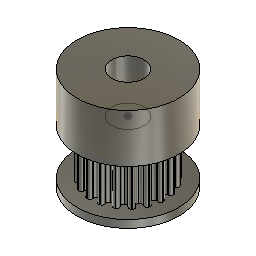
drive gear, 5mm shaft, 20 teeth v7 (Autodesk Fusion 360 design; units mm, degrees)
Autodesk Fusion 360 part; units mm, degrees
sketch "Sketch1" plane through (0, 0, 0) normal (0, 0, 1) x (1, 0, 0) in component "drive gear, 5mm shaft, 20 teeth"
  circle A0 centre (-19.8485, 10.6997) radius 8
  circle A1 centre (-19.8485, 10.6997) radius 2.5
  line L0 (-19.8485, 10.6997) -> (-14.5702, 12.4148) construction
  line L1 (-19.8485, 10.6997) -> (-14.7985, 10.6997) construction
  line L2 (-14.8275, 11.0683) -> (-14.8317, 11.1211)
  line L3 (-14.4955, 11.5475) -> (-14.3004, 11.5784)
  line L4 (-14.5702, 12.4148) -> (-14.5062, 12.4355)
  line L5 (-14.4288, 10.6997) -> (-14.2985, 10.6997)
  line L6 (-13.974, 12.0669) -> (-13.9936, 12.1485)
  arc A2 (-14.4955, 11.5475) -> (-14.8317, 11.1211) centre (-14.4329, 11.1525) ccw
  arc A3 (-14.8275, 11.0683) -> (-14.4288, 10.6997) centre (-14.4288, 11.0997) ccw
  arc A4 (-13.9936, 12.1485) -> (-14.5062, 12.4355) centre (-14.3826, 12.0551) ccw
  arc A5 (-14.3004, 11.5784) -> (-13.974, 12.0669) centre (-14.363, 11.9735) ccw
  line L7 (-14.694, 12.3745) -> (-14.5702, 12.4148)
  arc A6 (-15.1872, 12.6019) -> (-14.694, 12.3745) centre (-14.8176, 12.7549) ccw
  line L8 (-15.1872, 12.6019) -> (-15.2074, 12.6507)
  arc A7 (-15.0195, 13.1602) -> (-15.2074, 12.6507) centre (-14.8379, 12.8038) ccw
  line L9 (-15.0195, 13.1602) -> (-14.8435, 13.2499)
  arc A8 (-14.8435, 13.2499) -> (-14.684, 13.8153) centre (-15.0251, 13.6063) ccw
  line L10 (-14.684, 13.8153) -> (-14.7279, 13.8869)
  arc A9 (-14.7279, 13.8869) -> (-15.304, 14.0015) centre (-15.0689, 13.6779) ccw
  line L11 (-15.3585, 13.9619) -> (-15.304, 14.0015)
  line L12 (-15.4638, 13.8854) -> (-15.3585, 13.9619)
  arc A10 (-16.0031, 13.9492) -> (-15.4638, 13.8854) centre (-15.699, 14.209) ccw
  line L13 (-16.0031, 13.9492) -> (-16.0375, 13.9894)
  arc A11 (-16.0162, 14.5321) -> (-16.0375, 13.9894) centre (-15.7333, 14.2492) ccw
  line L14 (-16.0162, 14.5321) -> (-15.8765, 14.6717)
  arc A12 (-15.8765, 14.6717) -> (-15.8996, 15.2587) centre (-16.1593, 14.9546) ccw
  line L15 (-15.8996, 15.2587) -> (-15.9634, 15.3132)
  arc A13 (-15.9634, 15.3132) -> (-16.5468, 15.2442) centre (-16.2232, 15.0091) ccw
  line L16 (-16.5863, 15.1898) -> (-16.5468, 15.2442)
  line L17 (-16.6629, 15.0844) -> (-16.5863, 15.1898)
  arc A14 (-17.1955, 14.9784) -> (-16.6629, 15.0844) centre (-16.9865, 15.3195) ccw
  line L18 (-17.1955, 14.9784) -> (-17.2406, 15.0061)
  arc A15 (-17.388, 15.5287) -> (-17.2406, 15.0061) centre (-17.0316, 15.3471) ccw
  line L19 (-17.388, 15.5287) -> (-17.2983, 15.7047)
  arc A16 (-17.2983, 15.7047) -> (-17.5017, 16.2559) centre (-17.6547, 15.8863) ccw
  line L20 (-17.5017, 16.2559) -> (-17.5792, 16.288)
  arc A17 (-17.5792, 16.288) -> (-18.1127, 16.0421) centre (-17.7323, 15.9185) ccw
  line L21 (-18.1335, 15.9781) -> (-18.1127, 16.0421)
  line L22 (-18.1737, 15.8542) -> (-18.1335, 15.9781)
  arc A18 (-18.6475, 15.5889) -> (-18.1737, 15.8542) centre (-18.5541, 15.9778) ccw
  line L23 (-18.6475, 15.5889) -> (-18.699, 15.6012)
  arc A19 (-19.0007, 16.0527) -> (-18.699, 15.6012) centre (-18.6056, 15.9902) ccw
  line L24 (-19.0007, 16.0527) -> (-18.9698, 16.2478)
  arc A20 (-18.9698, 16.2478) -> (-19.3335, 16.7092) centre (-19.3649, 16.3104) ccw
  line L25 (-19.3335, 16.7092) -> (-19.4171, 16.7158)
  arc A21 (-19.4171, 16.7158) -> (-19.8485, 16.317) centre (-19.4485, 16.317) ccw
  line L26 (-19.8485, 16.2497) -> (-19.8485, 16.317)
  line L27 (-19.8485, 16.1195) -> (-19.8485, 16.2497)
  arc A22 (-20.2171, 15.7207) -> (-19.8485, 16.1195) centre (-20.2485, 16.1195) ccw
  line L28 (-20.2171, 15.7207) -> (-20.2699, 15.7165)
  arc A23 (-20.6964, 16.0527) -> (-20.2699, 15.7165) centre (-20.3013, 16.1153) ccw
  line L29 (-20.6964, 16.0527) -> (-20.7273, 16.2478)
  arc A24 (-20.7273, 16.2478) -> (-21.2157, 16.5742) centre (-21.1223, 16.1853) ccw
  line L30 (-21.2157, 16.5742) -> (-21.2973, 16.5546)
  arc A25 (-21.2973, 16.5546) -> (-21.5844, 16.0421) centre (-21.2039, 16.1657) ccw
  line L31 (-21.5636, 15.9781) -> (-21.5844, 16.0421)
  line L32 (-21.5233, 15.8542) -> (-21.5636, 15.9781)
  arc A26 (-21.7507, 15.361) -> (-21.5233, 15.8542) centre (-21.9037, 15.7306) ccw
  line L33 (-21.7507, 15.361) -> (-21.7996, 15.3408)
  arc A27 (-22.309, 15.5287) -> (-21.7996, 15.3408) centre (-21.9526, 15.7103) ccw
  line L34 (-22.309, 15.5287) -> (-22.3987, 15.7047)
  arc A28 (-22.3987, 15.7047) -> (-22.9641, 15.8642) centre (-22.7551, 15.5231) ccw
  line L35 (-22.9641, 15.8642) -> (-23.0357, 15.8204)
  arc A29 (-23.0357, 15.8204) -> (-23.1503, 15.2442) centre (-22.8267, 15.4793) ccw
  line L36 (-23.1107, 15.1898) -> (-23.1503, 15.2442)
  line L37 (-23.0342, 15.0844) -> (-23.1107, 15.1898)
  arc A30 (-23.098, 14.5451) -> (-23.0342, 15.0844) centre (-23.3578, 14.8493) ccw
  line L38 (-23.098, 14.5451) -> (-23.1382, 14.5107)
  arc A31 (-23.6809, 14.5321) -> (-23.1382, 14.5107) centre (-23.398, 14.8149) ccw
  line L39 (-23.6809, 14.5321) -> (-23.8205, 14.6717)
  arc A32 (-23.8205, 14.6717) -> (-24.4075, 14.6487) centre (-24.1034, 14.3889) ccw
  line L40 (-24.4075, 14.6487) -> (-24.462, 14.5848)
  arc A33 (-24.462, 14.5848) -> (-24.393, 14.0015) centre (-24.1579, 14.3251) ccw
  line L41 (-24.3386, 13.9619) -> (-24.393, 14.0015)
  line L42 (-24.2332, 13.8854) -> (-24.3386, 13.9619)
  arc A34 (-24.1272, 13.3528) -> (-24.2332, 13.8854) centre (-24.4683, 13.5618) ccw
  line L43 (-24.1272, 13.3528) -> (-24.1549, 13.3076)
  arc A35 (-24.6776, 13.1602) -> (-24.1549, 13.3076) centre (-24.496, 13.5166) ccw
  line L44 (-24.6776, 13.1602) -> (-24.8536, 13.2499)
  arc A36 (-24.8536, 13.2499) -> (-25.4047, 13.0466) centre (-25.0351, 12.8935) ccw
  line L45 (-25.4047, 13.0466) -> (-25.4368, 12.969)
  arc A37 (-25.4368, 12.969) -> (-25.1909, 12.4355) centre (-25.0673, 12.816) ccw
  line L46 (-25.1269, 12.4148) -> (-25.1909, 12.4355)
  line L47 (-25.003, 12.3745) -> (-25.1269, 12.4148)
  arc A38 (-24.7377, 11.9007) -> (-25.003, 12.3745) centre (-25.1266, 11.9941) ccw
  line L48 (-24.7377, 11.9007) -> (-24.75, 11.8492)
  arc A39 (-25.2015, 11.5475) -> (-24.75, 11.8492) centre (-25.139, 11.9426) ccw
  line L49 (-25.2015, 11.5475) -> (-25.3966, 11.5784)
  arc A40 (-25.3966, 11.5784) -> (-25.858, 11.2148) centre (-25.4592, 11.1834) ccw
  line L50 (-25.858, 11.2148) -> (-25.8646, 11.1311)
  arc A41 (-25.8646, 11.1311) -> (-25.4658, 10.6997) centre (-25.4658, 11.0997) ccw
  line L51 (-25.3985, 10.6997) -> (-25.4658, 10.6997)
  line L52 (-25.2683, 10.6997) -> (-25.3985, 10.6997)
  arc A42 (-24.8695, 10.3311) -> (-25.2683, 10.6997) centre (-25.2683, 10.2997) ccw
  line L53 (-24.8695, 10.3311) -> (-24.8654, 10.2783)
  arc A43 (-25.2015, 9.8519) -> (-24.8654, 10.2783) centre (-25.2641, 10.2469) ccw
  line L54 (-25.2015, 9.8519) -> (-25.3966, 9.821)
  arc A44 (-25.3966, 9.821) -> (-25.723, 9.3325) centre (-25.3341, 9.4259) ccw
  line L55 (-25.723, 9.3325) -> (-25.7034, 9.2509)
  arc A45 (-25.7034, 9.2509) -> (-25.1909, 8.9639) centre (-25.3145, 9.3443) ccw
  line L56 (-25.1269, 8.9847) -> (-25.1909, 8.9639)
  line L57 (-25.003, 9.0249) -> (-25.1269, 8.9847)
  arc A46 (-24.5099, 8.7976) -> (-25.003, 9.0249) centre (-24.8794, 8.6445) ccw
  line L58 (-24.5099, 8.7976) -> (-24.4896, 8.7487)
  arc A47 (-24.6776, 8.2392) -> (-24.4896, 8.7487) centre (-24.8592, 8.5956) ccw
  line L59 (-24.6776, 8.2392) -> (-24.8536, 8.1495)
  arc A48 (-24.8536, 8.1495) -> (-25.013, 7.5841) centre (-24.672, 7.7931) ccw
  line L60 (-25.013, 7.5841) -> (-24.9692, 7.5126)
  arc A49 (-24.9692, 7.5126) -> (-24.393, 7.398) centre (-24.6281, 7.7216) ccw
  line L61 (-24.3386, 7.4375) -> (-24.393, 7.398)
  line L62 (-24.2332, 7.5141) -> (-24.3386, 7.4375)
  arc A50 (-23.6939, 7.4502) -> (-24.2332, 7.5141) centre (-23.9981, 7.1904) ccw
  line L63 (-23.6939, 7.4502) -> (-23.6595, 7.41)
  arc A51 (-23.6809, 6.8674) -> (-23.6595, 7.41) centre (-23.9637, 7.1502) ccw
  line L64 (-23.6809, 6.8674) -> (-23.8205, 6.7277)
  arc A52 (-23.8205, 6.7277) -> (-23.7975, 6.1407) centre (-23.5377, 6.4448) ccw
  line L65 (-23.7975, 6.1407) -> (-23.7337, 6.0862)
  arc A53 (-23.7337, 6.0862) -> (-23.1503, 6.1552) centre (-23.4739, 6.3903) ccw
  line L66 (-23.1107, 6.2097) -> (-23.1503, 6.1552)
  line L67 (-23.0342, 6.315) -> (-23.1107, 6.2097)
  arc A54 (-22.5016, 6.421) -> (-23.0342, 6.315) centre (-22.7106, 6.0799) ccw
  line L68 (-22.5016, 6.421) -> (-22.4564, 6.3933)
  arc A55 (-22.309, 5.8707) -> (-22.4564, 6.3933) centre (-22.6654, 6.0523) ccw
  line L69 (-22.309, 5.8707) -> (-22.3987, 5.6947)
  arc A56 (-22.3987, 5.6947) -> (-22.1954, 5.1435) centre (-22.0423, 5.5131) ccw
  line L70 (-22.1954, 5.1435) -> (-22.1178, 5.1114)
  arc A57 (-22.1178, 5.1114) -> (-21.5844, 5.3574) centre (-21.9648, 5.481) ccw
  line L71 (-21.5636, 5.4213) -> (-21.5844, 5.3574)
  line L72 (-21.5233, 5.5452) -> (-21.5636, 5.4213)
  arc A58 (-21.0495, 5.8106) -> (-21.5233, 5.5452) centre (-21.1429, 5.4216) ccw
  line L73 (-21.0495, 5.8106) -> (-20.9981, 5.7982)
  arc A59 (-20.6964, 5.3467) -> (-20.9981, 5.7982) centre (-21.0914, 5.4092) ccw
  line L74 (-20.6964, 5.3467) -> (-20.7273, 5.1516)
  arc A60 (-20.7273, 5.1516) -> (-20.3636, 4.6902) centre (-20.3322, 5.089) ccw
  line L75 (-20.3636, 4.6902) -> (-20.2799, 4.6837)
  arc A61 (-20.2799, 4.6837) -> (-19.8485, 5.0824) centre (-20.2485, 5.0824) ccw
  line L76 (-19.8485, 5.1497) -> (-19.8485, 5.0824)
  line L77 (-19.8485, 5.2799) -> (-19.8485, 5.1497)
  arc A62 (-19.4799, 5.6787) -> (-19.8485, 5.2799) centre (-19.4485, 5.2799) ccw
  line L78 (-19.4799, 5.6787) -> (-19.4271, 5.6829)
  arc A63 (-19.0007, 5.3467) -> (-19.4271, 5.6829) centre (-19.3958, 5.2841) ccw
  line L79 (-19.0007, 5.3467) -> (-18.9698, 5.1516)
  arc A64 (-18.9698, 5.1516) -> (-18.4813, 4.8252) centre (-18.5747, 5.2142) ccw
  line L80 (-18.4813, 4.8252) -> (-18.3997, 4.8448)
  arc A65 (-18.3997, 4.8448) -> (-18.1127, 5.3574) centre (-18.4931, 5.2337) ccw
  line L81 (-18.1335, 5.4213) -> (-18.1127, 5.3574)
  line L82 (-18.1737, 5.5452) -> (-18.1335, 5.4213)
  arc A66 (-17.9464, 6.0384) -> (-18.1737, 5.5452) centre (-17.7933, 5.6688) ccw
  line L83 (-17.9464, 6.0384) -> (-17.8975, 6.0586)
  arc A67 (-17.388, 5.8707) -> (-17.8975, 6.0586) centre (-17.7444, 5.6891) ccw
  line L84 (-17.388, 5.8707) -> (-17.2983, 5.6947)
  arc A68 (-17.2983, 5.6947) -> (-16.7329, 5.5352) centre (-16.9419, 5.8763) ccw
  line L85 (-16.7329, 5.5352) -> (-16.6614, 5.5791)
  arc A69 (-16.6614, 5.5791) -> (-16.5468, 6.1552) centre (-16.8704, 5.9201) ccw
  line L86 (-16.5863, 6.2097) -> (-16.5468, 6.1552)
  line L87 (-16.6629, 6.315) -> (-16.5863, 6.2097)
  arc A70 (-16.599, 6.8543) -> (-16.6629, 6.315) centre (-16.3393, 6.5501) ccw
  line L88 (-16.599, 6.8543) -> (-16.5588, 6.8887)
  arc A71 (-16.0162, 6.8674) -> (-16.5588, 6.8887) centre (-16.299, 6.5845) ccw
  line L89 (-16.0162, 6.8674) -> (-15.8765, 6.7277)
  arc A72 (-15.8765, 6.7277) -> (-15.2895, 6.7508) centre (-15.5937, 7.0105) ccw
  line L90 (-15.2895, 6.7508) -> (-15.235, 6.8146)
  arc A73 (-15.235, 6.8146) -> (-15.304, 7.398) centre (-15.5392, 7.0743) ccw
  line L91 (-15.3585, 7.4375) -> (-15.304, 7.398)
  line L92 (-15.4638, 7.5141) -> (-15.3585, 7.4375)
  arc A74 (-15.5698, 8.0467) -> (-15.4638, 7.5141) centre (-15.2287, 7.8377) ccw
  line L93 (-15.5698, 8.0467) -> (-15.5421, 8.0918)
  arc A75 (-15.0195, 8.2392) -> (-15.5421, 8.0918) centre (-15.2011, 7.8828) ccw
  line L94 (-15.0195, 8.2392) -> (-14.8435, 8.1495)
  arc A76 (-14.8435, 8.1495) -> (-14.2923, 8.3528) centre (-14.6619, 8.5059) ccw
  line L95 (-14.2923, 8.3528) -> (-14.2602, 8.4304)
  arc A77 (-14.2602, 8.4304) -> (-14.5062, 8.9639) centre (-14.6298, 8.5834) ccw
  line L96 (-14.5702, 8.9847) -> (-14.5062, 8.9639)
  line L97 (-14.694, 9.0249) -> (-14.5702, 8.9847)
  arc A78 (-14.9594, 9.4987) -> (-14.694, 9.0249) centre (-14.5704, 9.4053) ccw
  line L98 (-14.9594, 9.4987) -> (-14.947, 9.5502)
  arc A79 (-14.4955, 9.8519) -> (-14.947, 9.5502) centre (-14.5581, 9.4568) ccw
  line L99 (-14.4955, 9.8519) -> (-14.3004, 9.821)
  arc A80 (-14.3004, 9.821) -> (-13.8391, 10.1847) centre (-14.2378, 10.216) ccw
  line L100 (-13.8391, 10.1847) -> (-13.8325, 10.2683)
  arc A81 (-13.8325, 10.2683) -> (-14.2312, 10.6997) centre (-14.2312, 10.2997) ccw
  line L101 (-14.2985, 10.6997) -> (-14.2312, 10.6997)
  dimension "d6_1_1" = 16
  dimension "d8_1_1" = 5
  dimension "d1_1" = 18
  dimension "d19_1" = 5.55
  dimension "d20_1" = 5.05
  dimension "d22_1" = 0.5
  dimension "d24_1" = 0.4
  dimension "d25_1" = 0.4
  dimension "d26_1" = 0.4
  dimension "d27_1" = 0.4
  dimension "d29_1" = 360
  constraint concentric A0 A1
  constraint horizontal L1
  constraint parallel L0 L4
  constraint coincident A0.centre A1.centre
  constraint parallel L1 L5
  constraint tangent L3 A2
  constraint tangent L2 A3
  constraint tangent L6 A4
  constraint tangent L3 A5
  constraint tangent L4 A4
  constraint tangent L6 A5
  constraint tangent L2 A2
  constraint tangent L5 A3
  measures "d6_1_1" diameter of A0
  measures "d8_1_1" diameter of A1
  measures "d1_1" angle of L0 L1
  measures "d19_1" distance of A0.centre L0.end
  measures "d20_1" distance of A0.centre L1.end
  measures "d22_1" distance of L1.end L5.end
  measures "d24_1" radius of A3
  measures "d25_1" radius of A2
  measures "d26_1" radius of A5
  measures "d27_1" radius of A4
extrude "Extrude1" add sketch "Sketch1" along normal mid plane 9.65 contours A0 | L2 L3 L4 L5 L6 A2 A3 A4 A5 L7 A6 L8 A7 L9 A8 L10 A9 L11 L12 A10 L13 A11 L14 A12 L15 A13 L16 L17 A14 L18 A15 L19 A16 L20 A17 L21 L22 A18 L23 A19 L24 A20 L25 A21 L26 L27 A22 L28 A23 L29 A24 L30 A25 L31 L32 A26 L33 A27 L34 A28 L35 A29 L36 L37 A30 L38 A31 L39 A32 L40 A33 L41 L42 A34 L43 A35 L44 A36 L45 A37 L46 L47 A38 L48 A39 L49 A40 L50 A41 L51 L52 A42 L53 A43 L54 A44 L55 A45 L56 L57 A46 L58 A47 L59 A48 L60 A49 L61 L62 A50 L63 A51 L64 A52 L65 A53 L66 L67 A54 L68 A55 L69 A56 L70 A57 L71 L72 A58 L73 A59 L74 A60 L75 A61 L76 L77 A62 L78 A63 L79 A64 L80 A65 L81 L82 A66 L83 A67 L84 A68 L85 A69 L86 L87 A70 L88 A71 L89 A72 L90 A73 L91 L92 A74 L93 A75 L94 A76 L95 A77 L96 L97 A78 L98 A79 L99 A80 L100 A81 L101 in component "drive gear, 5mm shaft, 20 teeth"
extrude "Extrude2" cut sketch "Sketch1" along normal mid plane 7.25 in component "drive gear, 5mm shaft, 20 teeth"
sketch "Sketch1 (2)" plane through (0, 0, 4.825) normal (0, 0, 1) x (-1, 0, 0)
  circle A0 centre (19.8485, -10.6997) radius 2.5
  circle A1 centre (19.8485, -10.6997) radius 8
  circle A2 centre (19.8485, -10.6997) radius 2.55
  dimension "d5" = 5.1
  constraint concentric A0 A2
  measures "d5" diameter of A2
extrude "Extrude3" add sketch "Sketch1 (2)" along normal blind 6.45 contours A1 in component "drive gear, 5mm shaft, 20 teeth"
component "drive gear, 5mm shaft, 20 teeth" placed x (1, 0, 0) y (0, 1, 0) z (0, 0, 1) at (0, 0, 0)
equation "d6_1_1 = flange_diameter_1_1"
equation "d8_1_1 = shaft_diameter_1_1"
equation "d9_1_1 = 2 * flange_thickness + belt_space_1_1"
equation "d11_1_1 = belt_space_1_1"
equation "d1_1 = ( 360 / number_of_teeth_1_1 ) * 1 deg"
equation "d3_1 = pulley_diameter_1_1 / 2 - 1 mm"
equation "d4_1 = d1_1 / 2"
equation "d19_1 = pulley_diameter_1_1 / 2 - 0.5 mm"
equation "d20_1 = pulley_diameter_1_1 / 2 - 1 mm"
equation "d25_1 = d24_1"
equation "d27_1 = d26_1"
equation "shaft_diameter_1_1 = 5 mm"
equation "flange_diameter_1_1 = 16 mm"
equation "pulley_diameter_1_1 = 12.1 mm"
equation "belt_space_1_1 = 7.25 mm"
equation "middle_height = 9 mm"
equation "number_of_teeth_1_1 = 20"
equation "overall_height_1_1 = 16.1 mm"
equation "d5 = shaft_diameter_1_1 + 0.1 mm"
equation "d6 = overall_height_1_1 - belt_space_1_1 - 2 * flange_thickness"
equation "flange_thickness = 1.2 mm"
named bodies: "drive gear, 5mm shaft, 20 teeth"
